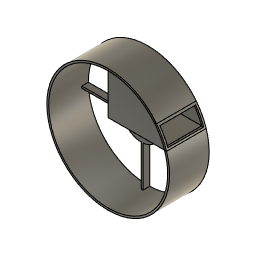
Petfeeder_internal (Autodesk Fusion 360 design; units mm, degrees)
Autodesk Fusion 360 part; units mm, degrees
sketch "Sketch1" plane through (0, 0, 0) normal (0, 1, 0) x (1, 0, 0)
  circle A0 centre (0, 0) radius 65
  circle A1 centre (0, 0) radius 63
  circle A2 centre (0, 0) radius 20
  line L0 (0, -20) -> (0, -63)
  line L1 (20, 0) -> (63, 0)
  line L2 (0, 0) -> (0, 2)
  line L3 (0, 20) -> (0, 63)
  line L4 (0, 0) -> (-2, 0)
  line L5 (-20, 0) -> (-63, 0)
  line L6 (-19.8997, 2) -> (-62.9682, 2)
  line L7 (-64.9692, 2) -> (-65, 2)
  line L8 (2, 19.8997) -> (2, 62.9682)
  line L9 (2, 64.9692) -> (2, 65)
  line L10 (19.8997, -2) -> (62.9682, -2)
  line L11 (64.9692, -2) -> (65, -2)
  line L12 (-2, -19.8997) -> (-2, -62.9682)
  line L13 (-2, -64.9692) -> (-2, -65)
  line L14 (0, -20) -> (59.7411, -20)
  line L15 (2, -22) -> (0, -22)
  line L16 (59.7411, -20) -> (61.8466, -20)
  line L17 (61.8466, -20) -> (61.8466, -40)
  line L18 (61.8466, -40) -> (48.6724, -40)
  dimension "d1" = 130
  dimension "d2" = -2
  dimension "d3" = 40
  dimension "d19" = 20
  constraint coincident A0.centre A1.centre
  constraint concentric A0 A2
  constraint vertical L0
  constraint coincident A2 L3.start
  constraint collinear L2 L3
  constraint coincident A2 L8.start
  constraint coincident A2 L1.start
  constraint coincident A2 L10.start
  constraint coincident A2 L6.start
  constraint coincident A2 L5.start
  constraint collinear L4 L5
  constraint coincident A1 L6.end
  constraint coincident A0 L7.start
  constraint collinear L6 L7
  constraint coincident A1 L5.end
  constraint coincident A1 L3.end
  constraint coincident A1 L8.end
  constraint coincident A0 L9.start
  constraint collinear L8 L9
  constraint coincident A1 L10.end
  constraint coincident A0 L11.start
  constraint collinear L10 L11
  constraint coincident A1 L1.end
  constraint coincident A2 L12.start
  constraint coincident A2 L0.start
  constraint coincident A1 L0.end
  constraint coincident A1 L12.end
  constraint coincident A0 L13.start
  constraint collinear L12 L13
  constraint tangent A2 L14
  constraint perpendicular L0 L14
  constraint coincident L0 L15.end
  constraint perpendicular L0 L15
  constraint coincident A1 L14.end
  constraint coincident A0 L16.end
  constraint parallel L14 L16
  constraint coincident A1 L18.end
  constraint perpendicular L17 L18
  measures "d1" diameter of A0
  measures "d3" diameter of A2
  measures "d19" distance of L16.end L17.end
extrude "Extrude1" add sketch "Sketch1" along normal blind 42 contours A0 A1 L16 L18 | A0 A1 L16 L18 | A1 A2 L1 L10 | A1 A2 L0 L12 | A2 | A1 A2 L3 L8 | A1 A2 L5 L6 makes body 1
sketch "Sketch2" plane through (0, 0, 0) normal (0, -1, 0) x (1, 0, 0)
  line L0 (20, 0) -> (63, 0)
  arc A0 (2, -62.9682) -> (63, 0) centre (0, 0) ccw
  line L1 (2, -62.9682) -> (2, -19.8997)
  arc A1 (2, -19.8997) -> (20, 0) centre (0, 0) ccw
  line L2 (-20, 0) -> (-63, 0)
  arc A2 (-2, 62.9682) -> (-63, 0) centre (0, 0) ccw
  line L3 (-2, 62.9682) -> (-2, 19.8997)
  arc A3 (-2, 19.8997) -> (-20, 0) centre (0, 0) ccw
  line L4 (0, -20) -> (0, -63)
  arc A4 (-62.9682, -2) -> (0, -63) centre (0, 0) ccw
  line L5 (-62.9682, -2) -> (-19.8997, -2)
  arc A5 (-19.8997, -2) -> (0, -20) centre (0, 0) ccw
  line L6 (0, 20) -> (0, 63)
  arc A6 (62.9682, 2) -> (0, 63) centre (0, 0) ccw
  line L7 (62.9682, 2) -> (19.8997, 2)
  arc A7 (19.8997, 2) -> (0, 20) centre (0, 0) ccw
  circle A8 centre (0, 0) radius 65
  circle A9 centre (0, 0) radius 63
  dimension "d9" = -2
extrude "Extrude2" cut sketch "Sketch2" against normal blind 35 contours L0 L1 A1 L2 L3 A3 L4 L5 A5 L6 L7 A7 A9 bodies 1
sketch "Sketch3" plane through (0, 42, 0) normal (0, 1, 0) x (-1, 0, 0)
  line L0 (-63, 0) -> (-20, 0)
  arc A0 (-20, 0) -> (-2, -19.8997) centre (0, 0) ccw
  line L1 (-2, -19.8997) -> (-2, -62.9682)
  arc A1 (-63, 0) -> (-2, -62.9682) centre (0, 0) ccw
  line L2 (63, 0) -> (20, 0)
  arc A2 (20, 0) -> (2, 19.8997) centre (0, 0) ccw
  line L3 (2, 19.8997) -> (2, 62.9682)
  arc A3 (63, 0) -> (2, 62.9682) centre (0, 0) ccw
  line L4 (0, -63) -> (0, -20)
  arc A4 (0, -20) -> (19.8997, -2) centre (0, 0) ccw
  line L5 (19.8997, -2) -> (62.9682, -2)
  arc A5 (0, -63) -> (62.9682, -2) centre (0, 0) ccw
  line L6 (0, 63) -> (0, 20)
  arc A6 (0, 20) -> (-19.8997, 2) centre (0, 0) ccw
  line L7 (-19.8997, 2) -> (-62.9682, 2)
  arc A7 (0, 63) -> (-62.9682, 2) centre (0, 0) ccw
  circle A8 centre (0, 0) radius 65
  circle A9 centre (0, 0) radius 10.425
  dimension "d12" = 20.85
  constraint concentric A0 A9
  measures "d12" diameter of A9
extrude "Extrude3" cut sketch "Sketch3" against normal blind 3 contours A9 bodies 1
sketch "Sketch4" plane through (0, 39, 0) normal (0, 1, 0) x (-1, 0, 0)
  circle A0 centre (0, 0) radius 10.425
  circle A1 centre (0, 0) radius 1.5
  dimension "d15" = 3
  constraint coincident A0.centre A1.centre
  measures "d15" diameter of A1
extrude "Extrude4" cut sketch "Sketch4" against normal blind 36 contours A1 bodies 1
sketch "Sketch5" plane through (0, 42, 0) normal (0, 1, 0) x (-1, 0, 0)
  circle A0 centre (0, 0) radius 10.425
  line L0 (-63, 0) -> (-20, 0)
  arc A1 (-20, 0) -> (-2, -19.8997) centre (0, 0) ccw
  line L1 (-2, -19.8997) -> (-2, -62.9682)
  arc A2 (-63, 0) -> (-2, -62.9682) centre (0, 0) ccw
  line L2 (63, 0) -> (20, 0)
  arc A3 (20, 0) -> (2, 19.8997) centre (0, 0) ccw
  line L3 (2, 19.8997) -> (2, 62.9682)
  arc A4 (63, 0) -> (2, 62.9682) centre (0, 0) ccw
  line L4 (0, -63) -> (0, -20)
  arc A5 (0, -20) -> (19.8997, -2) centre (0, 0) ccw
  line L5 (19.8997, -2) -> (62.9682, -2)
  arc A6 (0, -63) -> (62.9682, -2) centre (0, 0) ccw
  line L6 (0, 63) -> (0, 20)
  arc A7 (0, 20) -> (-19.8997, 2) centre (0, 0) ccw
  line L7 (-19.8997, 2) -> (-62.9682, 2)
  arc A8 (0, 63) -> (-62.9682, 2) centre (0, 0) ccw
  circle A9 centre (0, 0) radius 65
extrude "Extrude5" add sketch "Sketch1" along normal blind 42 separate body contours A0 L17 L18 | A0 A1 L16 L18 | A1 L0 L14 picked at (51.0242, -37.9332) makes body 2
shell "Shell1" thickness 2 removed faces 1 at (61.8466, 14, 26.6667) on bodies 2
sketch "Sketch6" plane through (61.8466, 0, 0) normal (1, 0, 0) x (0, 1, 0)
  line L0 (2, 38) -> (40, 38)
  line L1 (40, 38) -> (40, 22)
  line L2 (40, 22) -> (2, 22)
  line L3 (2, 22) -> (2, 38)
  line L4 (0, 40) -> (0, 20)
  line L5 (0, 20) -> (42, 20)
  line L6 (42, 20) -> (42, 40)
  line L7 (42, 40) -> (0, 40)
  line L8 (2, 38) -> (40, 38)
  line L9 (40, 38) -> (40, 22)
  line L10 (40, 22) -> (2, 22)
  line L11 (2, 22) -> (2, 38)
  constraint horizontal L8
  constraint vertical L9
  constraint horizontal L10
  constraint vertical L11
  constraint coincident L1.end L2.start
  constraint coincident L0.start L3.end
extrude "Extrude6" cut sketch "Sketch6" against normal blind 40 contours L0 L1 L2 L3 L8 L9 L10 L11 bodies 1
extrude "Extrude7" cut sketch "Sketch1" along normal blind 140 contours A0 L17 L18 bodies 2
